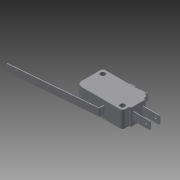
# Autodesk Inventor part: MICROSWITCH
Saved by Autodesk Inventor 2015 (Build 190159000, 159)
## iProperties
Created: 2015-02-07
Part Number: MICROSWITCH
Material: Generic
Document SubType Name: Sheet Metal
Designer: lucanao16
Density: 1 g/cm^3
Sheet Metal Rule: Default
Appearance: Default
Author: lucanao16
Autodesk Inventor part; units mm, degrees
ref_plane "YZ Plane" through (0, 0, 0) normal (1, 0, 0) x (0, 1, 0)
sketch "Sketch1" plane through (0, 0, 0) normal (0, 1, 0) x (-1, 0, 0)
  line L0 (0, 0) -> (27.686, 0)
  line L1 (27.686, 0) -> (27.686, -15.875)
  line L2 (27.686, -15.875) -> (0, -15.875)
  line L3 (0, -15.875) -> (0, 0)
  dimension "d0" = 27.686
  dimension "d1" = 15.875
  constraints: 8 end point, 2 parallel, 1 horizontal, 1 perpendicular
  measures "d0" distance of L1.end L2.end
  measures "d1" distance of L0.end L1.end
extrude "Extrusion1" add sketch "Sketch1" along normal blind 9.906
fillet "Fillet1" radius 3.175 2 edges at (-27.686, 4.953, 0) (0, 4.953, -15.875)
fillet "Fillet2" radius 1.5875 2 edges at (0, 4.953, 0) (-27.686, 4.953, -15.875)
sketch "Sketch3" plane through (0, 0, -12.7) normal (1, 0, 0) x (0, 0, -1)
  line L0 (0, 0) -> (-8.636, 0)
  line L1 (-8.636, 0) -> (-8.636, 9.906)
  line L2 (-8.636, 9.906) -> (0, 9.906)
  line L3 (0, 9.906) -> (0, 0)
  point P0 (-12.7, 0)
  dimension "d12" = 8.636
  constraints: 8 end point, 2 parallel, 1 horizontal, 1 perpendicular
  measures "d12" distance of L1.end L2.end
extrude "Extrusion2" add sketch "Sketch3" along normal blind 1.0414
fillet "Fillet3" radius 0.3969 2 edges at (1.0414, 4.953, -12.7) (1.0414, 4.953, -4.064)
sketch "Sketch2" plane through (0, 9.906, 0) normal (0, 1, 0) x (1, 0, 0)
  line L0 (0, 1.5875) -> (0, 12.7) projected
  line L1 (-3.175, 15.875) -> (-26.0985, 15.875) projected
  arc A0 (0.6445, 4.064) -> (1.0414, 4.4609) centre (0.6445, 4.4609) ccw projected
  line L2 (1.0414, 12.3031) -> (1.0414, 4.4609) projected
  arc A1 (1.0414, 12.3031) -> (0.6445, 12.7) centre (0.6445, 12.3031) ccw projected
  line L3 (0, 12.7) -> (0.6445, 12.7) projected
  arc A2 (0, 12.7) -> (-3.175, 15.875) centre (-3.175, 12.7) ccw projected
  line L4 (-3.175, 15.875) -> (-26.0985, 15.875) projected
  arc A3 (-26.0985, 15.875) -> (-27.686, 14.2875) centre (-26.0985, 14.2875) ccw projected
  line L5 (-27.686, 14.2875) -> (-27.686, 3.175) projected
  arc A4 (-27.686, 3.175) -> (-24.511, 0) centre (-24.511, 3.175) ccw projected
  line L6 (-24.511, 0) -> (-1.5875, 0) projected
  arc A5 (-1.5875, 0) -> (0, 1.5875) centre (-1.5875, 1.5875) ccw projected
  line L7 (0, 1.5875) -> (0, 4.064) projected
  line L8 (0, 4.064) -> (0.6445, 4.064) projected
  line L9 (-27.686, 14.2875) -> (-27.686, 3.175) projected
  circle A6 centre (-2.7305, 2.7305) radius 1.4605
  point P0 (0, 0)
  dimension "MinimumRemnant" = 6.096
  dimension "d33" = 2.7305
  dimension "d34" = 2.921
  dimension "d35" = 2.7305
  constraints: 1 centre point
  measures "d33" distance from line of L0 A6.centre
  measures "d34" diameter of A6
  measures "d35" distance from line of L6 A6.centre
extrude "Extrusion3" cut sketch "Sketch2" against normal blind 25.4 contours A6
sketch "Sketch4" plane through (0, 9.906, 0) normal (0, 1, 0) x (1, 0, 0)
  line L0 (-1.5875, 0) -> (-24.511, 0) projected
  line L1 (-26.0985, 15.875) -> (-3.175, 15.875) projected
  line L2 (-27.686, 3.175) -> (-27.686, 14.2875) projected
  circle A0 centre (-2.7305, 2.7305) radius 1.4605 projected
  arc A1 (0.6445, 4.064) -> (1.0414, 4.4609) centre (0.6445, 4.4609) ccw projected
  line L3 (1.0414, 12.3031) -> (1.0414, 4.4609) projected
  arc A2 (1.0414, 12.3031) -> (0.6445, 12.7) centre (0.6445, 12.3031) ccw projected
  line L4 (0, 12.7) -> (0.6445, 12.7) projected
  arc A3 (0, 12.7) -> (-3.175, 15.875) centre (-3.175, 12.7) ccw projected
  line L5 (-3.175, 15.875) -> (-26.0985, 15.875) projected
  arc A4 (-26.0985, 15.875) -> (-27.686, 14.2875) centre (-26.0985, 14.2875) ccw projected
  line L6 (-27.686, 14.2875) -> (-27.686, 3.175) projected
  arc A5 (-27.686, 3.175) -> (-24.511, 0) centre (-24.511, 3.175) ccw projected
  line L7 (-24.511, 0) -> (-1.5875, 0) projected
  arc A6 (-1.5875, 0) -> (0, 1.5875) centre (-1.5875, 1.5875) ccw projected
  line L8 (0, 1.5875) -> (0, 4.064) projected
  line L9 (0, 4.064) -> (0.6445, 4.064) projected
  circle A7 centre (-24.9555, 13.1445) radius 1.4605
  line L10 (-24.9555, 13.1445) -> (-27.686, 13.1445)
  line L11 (-24.9555, 14.605) -> (-24.9555, 15.875)
  point P0 (0, 0)
  dimension "d28" = 2.921
  dimension "d27" = 2.7305
  dimension "d29" = 1.27
  constraints: 4 end point, 2 perpendicular, 2 point on line, 1 vertical alignment, 2 other
  measures "d27" distance of L10.start L10.end
  measures "d29" distance of L11.start L11.end
extrude "Extrusion4" cut sketch "Sketch4" against normal blind 25.4 contours A7
sketch "Sketch5" plane through (-24.511, 0, 0) normal (0, 0, 1) x (1, 0, 0)
  line L0 (25.5524, 0) -> (25.5524, 9.906) projected
  line L1 (22.9235, 9.906) -> (22.9235, 0) projected
  line L2 (0, 9.906) -> (22.9235, 9.906) projected
  line L3 (0, 0) -> (0, 9.906) projected
  line L4 (22.9235, 0) -> (0, 0) projected
  line L5 (0, 9.906) -> (22.9235, 9.906) projected
  line L6 (9.8044, 0) -> (10.8204, 0)
  line L7 (10.8204, 0) -> (10.8204, 9.906)
  line L8 (10.8204, 9.906) -> (9.8044, 9.906)
  line L9 (9.8044, 9.906) -> (9.8044, 0)
  line L10 (10.8204, 8.128) -> (9.8044, 8.128)
  line L11 (9.8044, 8.128) -> (9.8044, 1.778)
  line L12 (9.8044, 1.778) -> (10.8204, 1.778)
  line L13 (10.8204, 1.778) -> (10.8204, 8.128)
  point P0 (24.511, 0)
  dimension "d37" = 1.016
  dimension "d38" = 9.8044
  dimension "d39" = 6.35
  dimension "d40" = 1.778
  dimension "d41" = 9.906
  constraints: 16 end point, 4 parallel, 4 point on line, 2 horizontal, 2 perpendicular
  measures "d37" distance of L8.end L7.end
  measures "d38" distance between parallel lines of L9 L3
  measures "d39" distance of L11.end L10.end
  measures "d40" distance between parallel lines of L2 L10
  measures "d41" distance between parallel lines of L2 L4
extrude "Extrusion5" add sketch "Sketch5" along normal blind 1.143 contours L7 L12 L9 L10
sketch "Sketch6" plane through (-24.511, 0, 1.143) normal (0, 0, 1) x (1, 0, 0)
  line L0 (10.8204, 8.128) -> (9.8044, 8.128) projected
  line L1 (9.8044, 8.128) -> (9.8044, 1.778) projected
  line L2 (9.8044, 1.778) -> (10.8204, 1.778) projected
  line L3 (10.8204, 1.778) -> (10.8204, 8.128) projected
  line L4 (10.3124, 1.778) -> (9.8044, 1.778)
  line L5 (9.8044, 1.778) -> (9.8044, 8.128)
  line L6 (9.8044, 8.128) -> (10.3124, 8.128)
  line L7 (10.3124, 8.128) -> (10.3124, 1.778)
  point P0 (24.511, 0)
  constraints: 8 end point, 2 parallel, 1 horizontal, 1 midpoint, 1 perpendicular
extrude "Extrusion6" add sketch "Sketch6" along normal blind 1.143 contours L7 L2 L1 L0
ref_plane "Work Plane1" through (-14.7066, 8.128, 2.286) normal (0.9925462, 0, -0.1218693) x (0, -1, 0)
sketch "Sketch7" plane through (-14.7066, 8.128, 2.286) normal (0.9925462, 0, -0.1218693) x (0, -1, 0)
  line L0 (6.35, 2.269) -> (0, 2.269) projected
  line L1 (6.35, 2.269) -> (6.35, 0) projected
  line L2 (0, 0) -> (6.35, 0) projected
  line L3 (0, 2.269) -> (0, 0) projected
  line L4 (6.35, -0.0619) -> (0, -0.0619) projected
  line L5 (6.35, 2.269) -> (6.35, 0) projected
  line L6 (0, -0.0619) -> (6.35, -0.0619)
  line L7 (6.35, -0.0619) -> (6.35, 0.4461)
  line L8 (6.35, 0.4461) -> (0, 0.4461)
  line L9 (0, 0.4461) -> (0, -0.0619)
  point P0 (8.128, 0.4767)
  dimension "d47" = 0.508
  constraints: 8 end point, 2 parallel, 1 horizontal, 1 perpendicular, 1 point on line
  measures "d47" distance of L7.end L6.end
extrude "Extrusion7" add sketch "Sketch7" against normal blind 8.89 contours L1 L2 L3 L8 | L7 L4 L9 L2
extrude "Extrusion8" add sketch "Sketch7" along normal blind 0.254 contours L1 L2 L3 L8 | L7 L4 L9 L2
sketch "Sketch8" plane through (-14.4545, 8.128, 2.255) normal (0.9925462, 0, -0.1218693) x (-0.1218693, 0, -0.9925462)
  line L0 (0.4461, -6.35) -> (0.4461, 0) projected
  line L1 (2.269, 0) -> (0.4461, 0) projected
  line L2 (2.269, -6.35) -> (2.269, 0) projected
  line L3 (2.269, -6.35) -> (0.4461, -6.35) projected
  line L4 (0.4461, 0) -> (0.4461, -6.35) projected
  line L5 (0.4461, -6.35) -> (0.4461, 0) projected
  line L6 (-0.0312, 0) -> (-0.0312, -6.35) projected
  line L7 (-0.0312, 0) -> (-0.0619, 0) projected
  line L8 (-0.0619, 0) -> (-0.0619, -6.35) projected
  line L9 (-0.0619, -6.35) -> (-0.0312, -6.35) projected
  line L10 (-0.0312, -6.35) -> (-0.0619, -6.35)
  line L11 (-0.0619, -6.35) -> (-0.0619, 0)
  line L12 (-0.0619, 0) -> (-0.0312, 0)
  line L13 (-0.0312, 0) -> (-0.0312, -6.35)
  point P0 (0.4767, -8.128)
  constraints: 8 end point, 2 parallel, 1 horizontal, 1 perpendicular
loft "Loft1" add section 1 edges at (-14.4507, 4.953, 2.286) (-14.4488, 8.128, 2.3012) (-14.4469, 4.953, 2.3165) (-14.4488, 1.778, 2.3012) section 2 edges at (-14.1986, 4.953, 1.143) (-14.1986, 8.128, 1.7145) (-14.1986, 4.953, 2.286) (-14.1986, 1.778, 1.7145)
fillet "Fillet4" radius 0.3969 1 edges at (-14.1986, 4.953, 2.286)
fillet "Fillet5" radius 0.2646 1 edges at (-14.7066, 4.953, 1.8366)
sketch "Sketch9" plane through (-23.5228, 1.778, 3.4309) normal (0.1218693, 0, 0.9925462) x (0.9925462, 0, -0.1218693)
  line L0 (9.0431, 6.35) -> (9.0431, 0) projected
  line L1 (0, 6.35) -> (9.0431, 6.35) projected
  line L2 (0, 0) -> (0, 6.35) projected
  line L3 (0, 0) -> (9.0431, 0) projected
  line L4 (6.35, 5.4864) -> (0, 5.4864)
  line L5 (0, 5.4864) -> (0, 0.8636)
  line L6 (0, 0.8636) -> (6.35, 0.8636)
  line L7 (6.35, 0.8636) -> (6.35, 5.4864)
  line L8 (0, 6.35) -> (0, 0) projected
  line L9 (0, 3.175) -> (2.54, 3.175)
  line L10 (2.54, 3.175) -> (3.81, 3.175)
  circle A0 centre (3.175, 3.175) radius 0.635
  line L11 (6.35, 5.4864) -> (6.35, 6.35)
  line L12 (0, 6.35) -> (9.0431, 6.35) projected
  line L13 (6.35, 0.8636) -> (6.35, 0)
  line L14 (8.7107, 0) -> (0, 0) projected
  point P0 (23.7656, -1.778)
  dimension "d58" = 6.35
  dimension "d59" = 4.6228
  dimension "d60" = 0
  dimension "d61" = 0.8636
  dimension "d62" = 0.8636
  dimension "d63" = 2.54
  dimension "d64" = 2.3114
  dimension "d65" = 1.27
  constraints: 16 end point, 3 perpendicular, 3 point on line, 2 horizontal, 2 midpoint, 2 parallel, 1 horizontal alignment, 2 other
  measures "d58" distance of L6.end L5.end
  measures "d59" distance of L5.end L4.end
  measures "d60" distance between parallel lines of L2 L5
  measures "d61" distance between parallel lines of L1 L4
  measures "d62" distance between parallel lines of L3 L6
  measures "d63" distance of L9.start L9.end
  measures "d64" distance between parallel lines of L9 L4
  measures "d65" distance of L9.end L10.end
extrude "Extrusion9" cut sketch "Sketch9" against normal blind 0.762 contours L11 L4 L2 L1 | L3 L2 L6 L13 | A0 L10 | L10 A0
fillet "Fillet6" radius 0.7937 2 edges at (-23.5537, 7.2644, 3.1788) (-23.5537, 2.6416, 3.1788)
sketch "Sketch10" plane through (0, 9.906, 0) normal (0, 1, 0) x (1, 0, 0)
  circle A0 centre (-24.9555, 13.1445) radius 1.4605 projected
  circle A1 centre (-2.7305, 2.7305) radius 1.4605 projected
  arc A2 (0.6445, 4.064) -> (1.0414, 4.4609) centre (0.6445, 4.4609) ccw projected
  line L0 (1.0414, 12.3031) -> (1.0414, 4.4609) projected
  arc A3 (1.0414, 12.3031) -> (0.6445, 12.7) centre (0.6445, 12.3031) ccw projected
  line L1 (0, 12.7) -> (0.6445, 12.7) projected
  arc A4 (0, 12.7) -> (-3.175, 15.875) centre (-3.175, 12.7) ccw projected
  line L2 (-3.175, 15.875) -> (-26.0985, 15.875) projected
  arc A5 (-26.0985, 15.875) -> (-27.686, 14.2875) centre (-26.0985, 14.2875) ccw projected
  line L3 (-27.686, 14.2875) -> (-27.686, 3.175) projected
  arc A6 (-27.686, 3.175) -> (-24.511, 0) centre (-24.511, 3.175) ccw projected
  line L4 (-24.511, 0) -> (-1.5875, 0) projected
  arc A7 (-1.5875, 0) -> (0, 1.5875) centre (-1.5875, 1.5875) ccw projected
  line L5 (0, 1.5875) -> (0, 4.064) projected
  line L6 (0, 4.064) -> (0.6445, 4.064) projected
  line L7 (-27.686, 3.175) -> (-27.686, 14.2875) projected
  point P0 (0, 0)
  point P1 (-13.843, 7.9375)
pattern_circular "Circular Pattern1" count 2 over 360 about axis through (-13.843, 9.906, -7.9375) along (0, 1, 0) of "Extrusion8", "Extrusion7", "Extrusion5", "Fillet6", "Extrusion9", "Fillet5", "Fillet4", "Loft1", "Extrusion6"
sketch "Sketch11" plane through (0, 9.906, 0) normal (0, 1, 0) x (1, 0, 0)
  line L0 (-1.5875, 0) -> (-32.214, 0)
  line L1 (-32.214, 0) -> (-32.214, -6.629)
  line L2 (-32.214, -6.629) -> (-1.5875, -6.629)
  line L3 (-1.5875, -6.629) -> (-1.5875, 0)
  point P0 (0, 0)
  constraints: 8 end point, 2 parallel, 1 horizontal, 1 perpendicular
extrude "Extrusion10" cut sketch "Sketch11" against normal blind 25.4
sketch "Sketch12" plane through (-24.511, 0, 0) normal (0, 0, 1) x (1, 0, 0)
  line L0 (-3.175, 9.906) -> (-3.175, 0) projected
  line L1 (-3.175, 0) -> (13.589, 0)
  line L2 (22.9235, 0) -> (0, 0) projected
  line L3 (0, 9.906) -> (22.9235, 9.906) projected
  line L4 (13.589, 0) -> (13.081, 0)
  line L5 (13.081, 0) -> (13.081, 9.906)
  line L6 (13.081, 9.906) -> (13.589, 9.906)
  line L7 (13.589, 9.906) -> (13.589, 0)
  line L8 (13.081, 2.8321) -> (13.589, 2.8321)
  line L9 (13.589, 2.8321) -> (13.589, 7.0739)
  line L10 (13.589, 7.0739) -> (13.081, 7.0739)
  line L11 (13.081, 7.0739) -> (13.081, 2.8321)
  point P0 (24.511, 0)
  dimension "d74" = 16.764
  dimension "d75" = 0.508
  dimension "d76" = 4.2418
  dimension "d77" = 2.8321
  dimension "d78" = 9.906
  constraints: 18 end point, 4 parallel, 4 point on line, 2 horizontal, 2 perpendicular
  measures "d74" distance of L0.end L1.end
  measures "d75" distance of L5.end L6.end
  measures "d76" distance of L9.end L8.end
  measures "d77" distance from line of L1.end L8
  measures "d78" distance between parallel lines of L2 L3
extrude "Extrusion11" add sketch "Sketch12" along normal blind 2.54 contours L5 L10 L7 L8
ref_plane "Work Plane3" through (-11.43, 7.0739, 2.54) normal (-0.9961947, 0, 0.0871557) x (0, -1, 0)
sketch "Sketch13" plane through (-11.43, 7.0739, 2.54) normal (-0.9961947, 0, 0.0871557) x (0, -1, 0)
  line L0 (4.2418, -2.5303) -> (0, -2.5303) projected
  line L1 (4.2418, -2.5303) -> (4.2418, 0) projected
  line L2 (0, 0) -> (4.2418, 0) projected
  line L3 (0, -2.5303) -> (0, 0) projected
  line L4 (0, 0) -> (4.2418, 0)
  line L5 (4.2418, 0) -> (4.2418, 0.508)
  line L6 (4.2418, 0.508) -> (0, 0.508)
  line L7 (0, 0.508) -> (0, 0)
  point P0 (7.0739, -1.5341)
  dimension "d82" = 0.508
  constraints: 8 end point, 2 parallel, 1 horizontal, 1 perpendicular
  measures "d82" distance of L5.end L4.end
extrude "Extrusion12" add sketch "Sketch13" along normal blind 50.8 contours L2 L7 L6 L5
sketch "Sketch14" plane through (-24.511, 0, 2.54) normal (0, 0, 1) x (1, 0, 0)
  line L0 (13.589, 7.0739) -> (13.081, 7.0739) projected
  line L1 (13.081, 7.0739) -> (13.081, 2.8321) projected
  line L2 (13.081, 2.8321) -> (13.589, 2.8321) projected
  line L3 (13.589, 2.8321) -> (13.589, 7.0739) projected
  point P0 (24.511, 0)
sketch "Sketch15" plane through (-11.43, 7.0739, 0) normal (0, 1, 0) x (1, 0, 0)
  arc A0 (0.0443, -3.0461) -> (0.508, -2.54) centre (0, -2.54) ccw
  line L0 (0.0443, -3.0461) -> (0, -2.54)
  line L1 (0, -2.54) -> (0.0443, -3.0461) projected
  line L2 (0, -2.54) -> (0.508, -2.54)
  line L3 (0, -2.54) -> (0.508, -2.54) projected
  point P0 (11.43, 0)
  constraints: 4 end point, 2 collinear, 2 point on circle, 1 centre point
extrude "Extrusion13" add sketch "Sketch15" against normal blind 4.2418
fillet "Fillet7" radius 0.2646 1 edges at (-11.43, 4.953, 2.54)
sketch "Sketch16" plane through (1.0414, 0, -12.7) normal (1, 0, 0) x (0, 0, -1)
  line L0 (-8.2391, 0) -> (-8.2391, 9.906) projected
  line L1 (-8.2391, 0) -> (-0.3969, 0) projected
  line L2 (-0.3969, 9.906) -> (-0.3969, 0) projected
  line L3 (-0.3969, 9.906) -> (-8.2391, 9.906) projected
  line L4 (-8.2391, 3.9086) -> (-0.3969, 3.9086)
  line L5 (-0.3969, 9.906) -> (-0.3969, 0) projected
  line L6 (-7.3692, 4.953) -> (-1.2732, 4.953)
  line L7 (-1.2732, 2.593) -> (-1.7304, 2.593)
  line L8 (-1.7304, 2.593) -> (-1.7304, 7.292)
  line L9 (-1.7304, 7.292) -> (-1.2732, 7.292)
  line L10 (-1.2732, 7.292) -> (-1.2732, 2.593)
  line L11 (-9.525, 0) -> (1.5875, 0) projected
  line L12 (-4.3212, 0) -> (-4.3212, 9.906)
  line L13 (1.5875, 9.906) -> (-9.525, 9.906) projected
  line L14 (-6.912, 2.593) -> (-6.912, 7.292)
  line L15 (-6.912, 7.292) -> (-7.3692, 7.292)
  line L16 (-7.3692, 7.292) -> (-7.3692, 2.593)
  line L17 (-7.3692, 2.593) -> (-6.912, 2.593)
  point P0 (-12.7, 0)
  dimension "d88" = 6.096
  dimension "d89" = 0.8763
  dimension "d90" = 7.8422
  dimension "d91" = 4.699
  dimension "d92" = 0.4572
  dimension "d93" = 0
  constraints: 22 end point, 4 horizontal, 4 point on line, 4 symmetric about line, 2 parallel, 2 perpendicular
  measures "d88" distance of L6.start L6.end
  measures "d89" distance from line of L2 L6.end
  measures "d90" distance of L0.start L1.end
  measures "d91" distance of L7.end L8.end
  measures "d92" distance of L8.end L9.end
  measures "d93" distance from line of L6.end L10
extrude "Extrusion14" add sketch "Sketch16" along normal blind 10.1346 contours L16 L6 L14 L4 | L4 L14 L17 L16 | L16 L15 L14 L6 | L8 L6 L10 L4 | L4 L10 L7 L8 | L8 L9 L10 L6
sketch "Sketch17" plane through (1.0414, 2.593, -5.3308) normal (0, 0, 1) x (1, 0, 0)
  line L0 (0, 0) -> (0, 4.699) projected
  line L1 (0, 0) -> (10.1346, 0) projected
  line L2 (10.1346, 4.699) -> (10.1346, 0) projected
  line L3 (0, 4.699) -> (10.1346, 4.699) projected
  circle A0 centre (7.5946, 2.3495) radius 0.635
  point P0 (-1.0414, -2.593)
  dimension "d96" = 1.27
  dimension "d97" = 2.54
  constraints: 1 centre point
  measures "d96" diameter of A0
  measures "d97" distance from line of L2 A0.centre
extrude "Extrusion15" cut sketch "Sketch17" against normal blind 10.1346 contours A0
chamfer "Chamfer1" distance 0.3969 angle 45 4 edges at (11.176, 7.292, -5.5594) (11.176, 2.593, -5.5594) (11.176, 2.593, -11.1982) (11.176, 7.292, -11.1982)
ref_plane "Work Plane2" through (-12.9794, 8.128, -18.161) normal (-0.9925462, 0, 0.1218693) x (0, -1, 0)
equation "\"MinimumRemnant\" = 2 * Thickness"
equation "\"BendRadius\" = Thickness"
equation "\"BendReliefWidth\" = Thickness"
equation "\"BendReliefDepth\" = 0.5 * Thickness"
equation "\"CornerReliefSize\" = 4 * Thickness"
equation "\"TransitionRadius\" = BendRadius"
equation "\"JacobiRadiusSize\" = BendRadius"
equation "\"GapSize\" = Thickness"
equation "\"Thickness\" = 3.048"
body "Solid1"
